Autodesk Fusion 360 part; units mm, degrees
(part 3 of 7)
sketch "Sketch73" plane through (0, 0, 10) normal (0, 0, -1) x (1, 0, 0)
  line L0 (-2, 4.1) -> (0, 4.1)
  line L1 (0, 4.1) -> (0, 5.7)
  arc A0 (8.6603, 8.7) -> (0, 5.7) centre (0, 19.7) ccw
  line L2 (8.6603, 8.7) -> (27.2, 8.7)
  line L3 (27.2, 8.7) -> (27.2, 33.9)
  line L4 (27.2, 33.9) -> (66.7, 33.9)
  line L5 (66.7, 33.9) -> (66.7, 8.7)
  line L6 (66.7, 8.7) -> (85.2397, 8.7)
  arc A1 (93.9, 5.7) -> (85.2397, 8.7) centre (93.9, 19.7) ccw
  line L7 (93.9, 5.7) -> (93.9, 4.1)
  line L8 (93.9, 4.1) -> (95.9, 4.1)
  line L9 (95.9, 4.1) -> (98.4, 4.1)
  line L10 (98.4, 4.1) -> (100.9, 4.1)
  line L11 (100.9, 4.1) -> (126.4, 4.1)
  line L12 (126.4, 4.1) -> (126.4, 25.3)
  arc A2 (126.4, 25.3) -> (116.4, 35.3) centre (116.4, 25.3) ccw
  line L13 (116.4, 35.3) -> (-22.5, 35.3)
  arc A3 (-22.5, 35.3) -> (-32.5, 25.3) centre (-22.5, 25.3) ccw
  line L14 (-32.5, 25.3) -> (-32.5, 4.1)
  line L15 (-32.5, 4.1) -> (-7, 4.1)
  line L16 (-7, 4.1) -> (-4.5, 4.1)
  line L17 (-4.5, 4.1) -> (-2, 4.1)
  line L18 (126.4, 25.3) -> (116.4, 25.3)
  line L19 (116.4, 35.3) -> (116.4, 25.3)
  line L20 (116.4, 25.3) -> (116.4, 4.1)
  line L21 (95.9, -0.9) -> (98.4, -0.9)
  line L22 (95.9, -0.9) -> (113.9, -0.9)
  line L23 (116.4, 2) -> (116.4, 1.2)
  line L24 (118.9, 1.6) -> (118.9, 4.1)
  line L25 (113.9, 1.6) -> (113.9, 4.1)
  line L26 (116.4, 2) -> (116.4, 1.6)
  circle A4 centre (116.4, 1.6) radius 0.4
  circle A5 centre (116.4, 25.3) radius 0.4
  arc A6 (113.9, 1.6) -> (118.9, 1.6) centre (116.4, 1.6) ccw
  circle A7 centre (116.4, 25.3) radius 2.5
  circle A8 centre (116.4, 1.6) radius 2.5
  line L27 (27.2, 4.1) -> (66.7, 4.1)
  line L28 (46.95, 4.1) -> (46.95, -10) construction
  line L29 (46.95, 4.1) -> (46.95, -10) construction
  circle A9 centre (-22.5, 1.6) radius 2.5
  line L30 (-25, 1.6) -> (-25, 4.1)
  line L31 (-7, 4.1) -> (-32.5, 4.1)
  circle A10 centre (-22.5, 25.3) radius 2.5
  line L32 (-20, 1.6) -> (-20, 4.1)
  circle A11 centre (-22.5, 25.3) radius 0.4
  circle A12 centre (-22.5, 1.6) radius 0.4
  point P0 (95.9, -0.9)
  dimension "d491" = 0.8
  dimension "d492" = 0.8
  dimension "d493" = 5
  dimension "d496" = 0.8
  dimension "d497" = 0.8
  constraint coincident L12.end A2.start
  constraint coincident A2.centre L18.end
  constraint coincident A2.end L13.start
  constraint coincident L11 L20.end
  constraint perpendicular L11 L20
  constraint coincident P0 L21.start
  constraint parallel L21 L22
  constraint perpendicular L22 L23
  constraint coincident L11 L24.end
  constraint perpendicular L11 L24
  constraint coincident L11 L25.end
  constraint perpendicular L11 L25
  constraint coincident L26.end A4.centre
  constraint concentric A4 A6
  constraint coincident A4 L23.start
  constraint coincident L23 L26.end
  constraint coincident A4 L23.end
  constraint concentric A6 A8
  constraint coincident L20.end A8
  constraint midpoint L27 L28.start
  constraint perpendicular L2 L28
  constraint symmetric L10.end L28 L15.end
  constraint symmetric L11.end L28 L14.end
  constraint symmetric L24.end L28 L30.end
  constraint symmetric L25.end L28 L32.end
  constraint symmetric L24.start L28 L30.start
  constraint symmetric L25.start L28 L32.start
  constraint symmetric A7 L28 A10
  constraint symmetric A8 L28 A9
  constraint symmetric L29.start L28 L28.start
  constraint symmetric L29.end L28 L28.end
  constraint concentric A10 A11
  constraint concentric A9 A12
  measures "d491" diameter of A4
  measures "d492" diameter of A5
  measures "d493" diameter of A7
  measures "d496" diameter of A11
  measures "d497" diameter of A12
extrude "Extrude58" add sketch "Sketch73" against normal blind 4.6 contours L15 A9 L31 L32 | L15 A9 L30 L31 | A9 | L11 L24 A8 | L11 L25 A8 | A6 A8 | A12 bodies 3
extrude "Extrude59" add sketch "Sketch73" along normal blind 18.4 contours A9 | L18 L19 A5 A7 | L19 L20 A5 A7 | L18 L20 A5 A7 | A6 A8 | A10 bodies 3
sketch "Sketch74" plane through (0, 0, 10) normal (0, 0, -1) x (1, 0, 0)
  circle A0 centre (-22.5, 25.3) radius 2.5
  arc A1 (-20, 1.6) -> (-25, 1.6) centre (-22.5, 1.6) ccw
  line L0 (-20, 1.6) -> (-20, 4.1)
  line L1 (-20, 4.1) -> (-7, 4.1)
  line L2 (-7, 4.1) -> (-4.5, 4.1)
  line L3 (-4.5, 4.1) -> (-2, 4.1)
  line L4 (-2, 4.1) -> (0, 4.1)
  line L5 (0, 4.1) -> (0, 5.7)
  arc A2 (8.6603, 8.7) -> (0, 5.7) centre (0, 19.7) ccw
  line L6 (8.6603, 8.7) -> (27.2, 8.7)
  line L7 (27.2, 8.7) -> (27.2, 33.9)
  line L8 (27.2, 33.9) -> (66.7, 33.9)
  line L9 (66.7, 33.9) -> (66.7, 8.7)
  line L10 (66.7, 8.7) -> (85.2397, 8.7)
  arc A3 (93.9, 5.7) -> (85.2397, 8.7) centre (93.9, 19.7) ccw
  line L11 (93.9, 5.7) -> (93.9, 4.1)
  line L12 (93.9, 4.1) -> (95.9, 4.1)
  line L13 (95.9, 4.1) -> (98.4, 4.1)
  line L14 (98.4, 4.1) -> (100.9, 4.1)
  line L15 (100.9, 4.1) -> (113.9, 4.1)
  line L16 (113.9, 4.1) -> (113.9, 1.6)
  arc A4 (118.9, 1.6) -> (113.9, 1.6) centre (116.4, 1.6) ccw
  line L17 (118.9, 1.6) -> (118.9, 4.1)
  line L18 (118.9, 4.1) -> (126.4, 4.1)
  line L19 (126.4, 4.1) -> (126.4, 25.3)
  arc A5 (126.4, 25.3) -> (116.4, 35.3) centre (116.4, 25.3) ccw
  line L20 (116.4, 35.3) -> (-22.5, 35.3)
  arc A6 (-22.5, 35.3) -> (-32.5, 25.3) centre (-22.5, 25.3) ccw
  line L21 (-32.5, 25.3) -> (-32.5, 4.1)
  line L22 (-32.5, 4.1) -> (-25, 4.1)
  line L23 (-25, 4.1) -> (-25, 1.6)
  circle A7 centre (116.4, 25.3) radius 2.5
  line L24 (79.9, 19.7) -> (79.9, 15.7)
  line L25 (79.9, 19.7) -> (79.9, 23.7)
  line L26 (79.9, 19.7) -> (66.7, 19.7)
  line L27 (66.7, 19.7) -> (66.7, 15.7)
  line L28 (66.7, 19.7) -> (66.7, 23.7)
  line L29 (66.7, 15.7) -> (81.7498, 15.7)
  line L30 (66.7, 23.7) -> (82, 23.7)
  line L31 (82, 23.7) -> (79.9, 23.7)
  line L32 (79.9, 23.7) -> (12.6632, 23.7)
  line L33 (12.6632, 15.7) -> (79.9, 15.7)
  line L34 (12.6632, 15.7) -> (9.5, 15.7)
  line L35 (9.5, 15.7) -> (9.5, 23.7)
  line L36 (9.5, 23.7) -> (12.6632, 23.7)
  line L37 (81.7498, 15.7) -> (83.7784, 15.7)
  line L38 (83.7784, 15.7) -> (83.7784, 23.7)
  line L39 (83.7784, 23.7) -> (82, 23.7)
  point P0 (79.9, 19.7)
  dimension "d500" = 4
  dimension "d501" = 4
  dimension "d502" = 4
  dimension "d503" = 4
  dimension "d504" = 180
  dimension "d505" = 8
  constraint coincident P0 L24.start
  constraint vertical L24
  constraint parallel L24 L25
  constraint horizontal L26
  constraint coincident L9 L26.end
  constraint perpendicular L26 L27
  constraint perpendicular L26 L28
  constraint perpendicular L24 L29
  constraint perpendicular L9 L30
  constraint perpendicular L32 L35
  constraint parallel L29 L37
  constraint perpendicular L30 L38
  constraint perpendicular L38 L39
  measures "d500" distance of P0 L24.end
  measures "d501" distance of P0 L25.end
  measures "d502" distance of L26.end L27.end
  measures "d503" distance of L26.end L28.end
  measures "d504" angle of L31 L32
  measures "d505" distance of L32.end L33.start
extrude "Extrude60" cut sketch "Sketch74" against normal blind 4.6 contours A2 L7 L32 L33 | A2 L32 L33 L34 L35 L36 | L9 L25 L26 L28 L30 L32 | L9 L24 L26 L27 L29 L33 | A3 L25 L30 L31 | A3 L24 L29 | A3 L29 L30 L31 L37 L38 L39 bodies 3
sketch "Sketch76" plane through (0, 0, 14.6) normal (0, 0, -1) x (1, 0, 0)
  line L0 (113.9, 1.6) -> (113.9, 4.1)
  line L1 (113.9, 4.1) -> (100.9, 4.1)
  line L2 (100.9, 4.1) -> (100.9, 1.6)
  arc A0 (98.4, -0.9) -> (100.9, 1.6) centre (98.4, 1.6) ccw
  line L3 (98.4, -0.9) -> (95.9, -0.9)
  line L4 (95.9, -0.9) -> (95.9, -77.2)
  line L5 (95.9, -77.2) -> (75.9, -77.2)
  line L6 (75.9, -77.2) -> (75.9, -85.1)
  line L7 (75.9, -85.1) -> (106.4, -85.1)
  arc A1 (106.4, -85.1) -> (126.4, -65.1) centre (106.4, -65.1) ccw
  line L8 (126.4, -65.1) -> (126.4, 4.1)
  line L9 (126.4, 4.1) -> (118.9, 4.1)
  line L10 (118.9, 4.1) -> (118.9, 1.6)
  arc A2 (113.9, 1.6) -> (118.9, 1.6) centre (116.4, 1.6) ccw
  line L11 (107.65, -43.95) -> (107.65, -38.95)
  line L12 (107.65, -38.95) -> (112.65, -38.95)
  line L13 (112.65, -38.95) -> (112.65, -43.95)
  line L14 (112.65, -43.95) -> (107.65, -43.95)
  circle A3 centre (117.6453, -56.4453) radius 2.85
  circle A4 centre (102.6547, -56.4453) radius 2.85
  line L15 (113.3329, -38.8299) -> (112.9477, -38.4448)
  line L16 (112.9477, -38.4448) -> (114.6448, -36.7477)
  line L17 (114.6448, -36.7477) -> (115.0299, -37.1329)
  arc A5 (122.2, -39.2591) -> (115.0299, -37.1329) centre (117.65, -41.45) ccw
  line L18 (122.2, -39.2591) -> (122.2, -43.6409)
  arc A6 (113.1, -43.6409) -> (122.2, -43.6409) centre (117.65, -41.45) ccw
  line L19 (113.1, -43.6409) -> (113.1, -39.2591)
  arc A7 (113.3329, -38.8299) -> (113.1, -39.2591) centre (117.65, -41.45) ccw
  line L20 (106.9671, -44.0701) -> (107.3523, -44.4552)
  line L21 (107.3523, -44.4552) -> (105.6552, -46.1523)
  line L22 (105.6552, -46.1523) -> (105.2701, -45.7671)
  arc A8 (98.115, -43.6717) -> (105.2701, -45.7671) centre (102.65, -41.45) ccw
  line L23 (98.115, -43.6717) -> (98.0852, -39.29)
  arc A9 (107.185, -39.2283) -> (98.0852, -39.29) centre (102.65, -41.45) ccw
  line L24 (107.185, -39.2283) -> (107.2148, -43.61)
  arc A10 (106.9671, -44.0701) -> (107.2148, -43.61) centre (102.65, -41.45) ccw
  line L25 (112.7701, -44.6329) -> (113.1552, -44.2477)
  line L26 (113.1552, -44.2477) -> (114.8523, -45.9448)
  line L27 (114.8523, -45.9448) -> (114.4671, -46.3299)
  arc A11 (112.3364, -53.5022) -> (114.4671, -46.3299) centre (110.15, -48.95) ccw
  line L28 (112.3364, -53.5022) -> (112.3364, -53.5)
  line L29 (112.3364, -53.5) -> (107.9591, -53.5)
  arc A12 (107.9591, -44.4) -> (107.9591, -53.5) centre (110.15, -48.95) ccw
  line L30 (107.9591, -44.4) -> (112.3409, -44.4)
  arc A13 (112.7701, -44.6329) -> (112.3409, -44.4) centre (110.15, -48.95) ccw
  line L31 (107.5299, -38.2671) -> (107.1448, -38.6523)
  line L32 (107.1448, -38.6523) -> (105.4477, -36.9552)
  line L33 (105.4477, -36.9552) -> (105.8329, -36.5701)
  arc A14 (107.9591, -29.4) -> (105.8329, -36.5701) centre (110.15, -33.95) ccw
  line L34 (107.9591, -29.4) -> (112.3409, -29.4)
  arc A15 (112.3409, -38.5) -> (112.3409, -29.4) centre (110.15, -33.95) ccw
  line L35 (112.3409, -38.5) -> (107.9591, -38.5)
  arc A16 (107.5299, -38.2671) -> (107.9591, -38.5) centre (110.15, -33.95) ccw
  circle A17 centre (110.15, -62.1) radius 2.5
  circle A18 centre (110.2363, -20.8316) radius 2.5
  circle A19 centre (117.6453, -56.4453) radius 5
  circle A20 centre (102.6547, -56.4453) radius 5
  dimension "d509" = 10
  dimension "d510" = 10
  constraint concentric A3 A19
  constraint concentric A4 A20
  measures "d509" diameter of A19
  measures "d510" diameter of A20
extrude "Extrude61" cut sketch "Sketch76" against normal blind 0.5 contours A19 | A20 bodies 3
sketch "Sketch77" plane through (0, 0, 10) normal (0, 0, -1) x (1, 0, 0)
  line L0 (66.7, 23.7) -> (80.4836, 23.7)
  arc A0 (93.9, 5.7) -> (80.4836, 23.7) centre (93.9, 19.7) ccw
  line L1 (93.9, 5.7) -> (93.9, 4.1)
  line L2 (93.9, 4.1) -> (95.9, 4.1)
  line L3 (95.9, 4.1) -> (98.4, 4.1)
  line L4 (98.4, 4.1) -> (100.9, 4.1)
  line L5 (100.9, 4.1) -> (113.9, 4.1)
  line L6 (113.9, 4.1) -> (113.9, 1.6)
  arc A1 (118.9, 1.6) -> (113.9, 1.6) centre (116.4, 1.6) ccw
  line L7 (118.9, 1.6) -> (118.9, 4.1)
  line L8 (118.9, 4.1) -> (126.4, 4.1)
  line L9 (126.4, 4.1) -> (126.4, 25.3)
  arc A2 (126.4, 25.3) -> (116.4, 35.3) centre (116.4, 25.3) ccw
  line L10 (116.4, 35.3) -> (-22.5, 35.3)
  arc A3 (-22.5, 35.3) -> (-32.5, 25.3) centre (-22.5, 25.3) ccw
  line L11 (-32.5, 25.3) -> (-32.5, 4.1)
  line L12 (-32.5, 4.1) -> (-25, 4.1)
  line L13 (-25, 4.1) -> (-25, 1.6)
  arc A4 (-20, 1.6) -> (-25, 1.6) centre (-22.5, 1.6) ccw
  line L14 (-20, 1.6) -> (-20, 4.1)
  line L15 (-20, 4.1) -> (-7, 4.1)
  line L16 (-7, 4.1) -> (-4.5, 4.1)
  line L17 (-4.5, 4.1) -> (-2, 4.1)
  line L18 (-2, 4.1) -> (0, 4.1)
  line L19 (0, 4.1) -> (0, 5.7)
  arc A5 (13.4164, 23.7) -> (0, 5.7) centre (0, 19.7) ccw
  line L20 (13.4164, 23.7) -> (27.2, 23.7)
  line L21 (27.2, 23.7) -> (27.2, 33.9)
  line L22 (27.2, 33.9) -> (66.7, 33.9)
  line L23 (66.7, 33.9) -> (66.7, 23.7)
  circle A6 centre (-22.5, 25.3) radius 2.5
  circle A7 centre (116.4, 25.3) radius 2.5
  line L24 (-22.5, 1.6) -> (-22.5, 25.3)
  line L25 (-22.5, 24.9) -> (-23, 24.9)
  line L26 (-23, 24.9) -> (-22, 24.9)
  line L27 (-22.5, 2) -> (-23, 2)
  line L28 (-22.5, 2) -> (-22, 2)
  line L29 (-22, 2) -> (-23, 2)
  line L30 (-23, 2) -> (-23, 24.9)
  line L31 (-23, 24.9) -> (-22, 24.9)
  line L32 (-22, 24.9) -> (-22, 2)
  line L33 (27.2, 4.5) -> (66.7, 4.5)
  line L34 (27.2, 4.1) -> (66.7, 4.1)
  line L35 (46.95, 4.5) -> (46.95, -16.4696) construction
  line L36 (116.4, 2) -> (116.9, 2)
  line L37 (116.9, 2) -> (116.9, 24.9)
  line L38 (116.4, 2) -> (115.9, 2)
  line L39 (116.9, 24.9) -> (115.9, 24.9)
  line L40 (115.9, 24.9) -> (115.9, 2)
  dimension "d513" = 1
  dimension "d514" = 0.5
  constraint coincident A4.centre L24.start
  constraint coincident A3.centre A6.centre
  constraint coincident L24 L25.start
  constraint perpendicular L24 L25
  constraint horizontal L26
  constraint coincident L24 L27.start
  constraint perpendicular L24 L27
  constraint perpendicular L24 L28
  constraint horizontal L29
  constraint vertical L30
  constraint horizontal L31
  constraint vertical L32
  constraint midpoint L33 L35.start
  constraint perpendicular L34 L35
  constraint symmetric L25.end L35 L37.end
  constraint symmetric L27.start L35 L36.start
  constraint symmetric L27.end L35 L36.end
  constraint symmetric L28.end L35 L38.end
  constraint symmetric L26.end L35 L39.end
  measures "d513" distance of L25.end L26.end
  measures "d514" distance of L27.start L27.end
extrude "Extrude63" add sketch "Sketch77" along normal blind 4 contours A1 A7 L37 L40 | A4 A6 L24 L32 | A4 A6 L24 L30 bodies 3
sketch "Sketch78" plane through (0, 0, 14.6) normal (0, 0, -1) x (1, 0, 0)
  line L0 (-25, 1.6) -> (-25, 4.1)
  line L1 (-25, 4.1) -> (-32.5, 4.1)
  line L2 (-32.5, 4.1) -> (-32.5, -25.2)
  line L3 (-32.5, -25.2) -> (-32.5, -65.1)
  arc A0 (-32.5, -65.1) -> (-12.5, -85.1) centre (-12.5, -65.1) ccw
  line L4 (-12.5, -85.1) -> (-2, -85.1)
  line L5 (-2, -85.1) -> (-2, -0.9)
  line L6 (-2, -0.9) -> (-4.5, -0.9)
  arc A1 (-7, 1.6) -> (-4.5, -0.9) centre (-4.5, 1.6) ccw
  line L7 (-7, 1.6) -> (-7, 4.1)
  line L8 (-7, 4.1) -> (-20, 4.1)
  line L9 (-20, 4.1) -> (-20, 1.6)
  arc A2 (-25, 1.6) -> (-20, 1.6) centre (-22.5, 1.6) ccw
  arc A3 (-9.5307, -48.3426) -> (-9.5307, -34.5574) centre (-10.1676, -41.45) ccw
  arc A4 (-22.9827, -48.1827) -> (-9.5307, -48.3426) centre (-16.25, -47.7) ccw
  arc A5 (-22.9827, -34.7173) -> (-22.9827, -48.1827) centre (-22.5, -41.45) ccw
  arc A6 (-9.5307, -34.5574) -> (-22.9827, -34.7173) centre (-16.25, -35.2) ccw
  circle A7 centre (-16.25, -62.1) radius 2.5
  circle A8 centre (-16.1626, -20.3028) radius 2.5
  circle A9 centre (-22.5, 1.6) radius 0.4
  circle A10 centre (-22.5, 1.6) radius 0.4
  circle A11 centre (-4.5, 1.6) radius 0.4
  line L10 (-22.5, 1.2) -> (-4.5, 1.2)
  line L11 (-4.5, 2) -> (-22.5, 2)
  line L12 (-4.5, 1.2) -> (-4.5, 2)
  line L13 (-22.5, 1.2) -> (-22.5, 2)
  line L14 (46.95, 4.5) -> (46.95, -16.4696)
  line L15 (98.4, 2) -> (116.4, 2)
  line L16 (98.4, 1.2) -> (98.4, 2)
  line L17 (116.4, 1.2) -> (98.4, 1.2)
  line L18 (116.4, 1.2) -> (116.4, 2)
  circle A12 centre (-22.5, 1.6) radius 0.4
  circle A13 centre (-4.5, 1.6) radius 0.4
  circle A14 centre (98.4, 1.6) radius 0.4
  circle A15 centre (98.4, 1.6) radius 0.4
  circle A16 centre (116.4, 1.6) radius 0.4
  point P0 (-4.9, 1.6)
  point P1 (116.4, 1.6)
  constraint coincident A9 L10.start
  constraint coincident A10 L10.start
  constraint coincident A11 L10.end
  constraint coincident A11 L11.start
  constraint coincident A9 L11.end
  constraint perpendicular L10 L12
  constraint perpendicular L11 L13
  constraint symmetric L10.start L14 L17.start
  constraint symmetric L10.end L14 L16.start
  constraint symmetric L11.start L14 L15.start
  constraint symmetric L11.end L14 L15.end
  constraint concentric A10 A12
  constraint concentric A11 A13
  constraint coincident A13 P0
  constraint concentric A14 A15
  constraint coincident P1 A16.centre
extrude "Extrude64" add sketch "Sketch78" along normal blind 8.6 contours A1 L7 L9 A2 L10 L11 | L15 L17 A14 A15 A16 bodies 3
extrude "Extrude65" add 2 faces at (-15.6667, -2.7, 14.6) (109.5667, -2.7, 14.6) along direction (0, 0, -1) blind 4.6 on bodies 3 bodies 3
sketch "Sketch79" plane through (0, 0, 10) normal (0, 0, -1) x (1, 0, 0)
  arc A0 (70.9, -81.15) -> (75.9, -81.15) centre (73.4, -81.15) ccw
  line L0 (70.9, -81.15) -> (70.9, -77.2)
  line L1 (70.9, -77.2) -> (47.4908, -77.2)
  arc A1 (46.4092, -77.2) -> (47.4908, -77.2) centre (46.95, -80.1) ccw
  line L2 (46.4092, -77.2) -> (10.5, -77.2)
  line L3 (10.5, -77.2) -> (10.5, -81.15)
  arc A2 (5.5, -81.15) -> (10.5, -81.15) centre (8, -81.15) ccw
  line L4 (5.5, -81.15) -> (5.5, -77.2)
  line L5 (5.5, -77.2) -> (-2, -77.2)
  line L6 (-2, -77.2) -> (-2, -85.1)
  line L7 (-2, -85.1) -> (75.9, -85.1)
  line L8 (75.9, -85.1) -> (75.9, -81.15)
  line L9 (46.95, -80.1) -> (73.4, -80.1)
  line L10 (46.95, -80.1) -> (23, -80.1)
  line L11 (73.4, -80.1) -> (73.4, -81.15)
  line L12 (20.5, -80.75) -> (20.5, -81.15)
  line L13 (20.5, -81.15) -> (20.1, -81.15)
  line L14 (20.5, -81.15) -> (20.9, -81.15)
  line L15 (20.5, -81.15) -> (20.1, -81.15)
  line L16 (23, -81.15) -> (23, -77.2)
  line L17 (18, -81.15) -> (18, -77.2)
  line L18 (18, -77.2) -> (23, -77.2)
  circle A3 centre (20.5, -81.15) radius 0.4
  line L19 (8, -81.15) -> (18, -81.15)
  line L20 (20.1, -81.15) -> (20.5, -81.15)
  arc A4 (18, -81.15) -> (23, -81.15) centre (20.5, -81.15) ccw
  dimension "d527" = 2.5
  dimension "d528" = 2.5
  dimension "d529" = 0.8
  constraint coincident A1.centre L9.start
  constraint horizontal L9
  constraint parallel L9 L10
  constraint coincident A0.centre L11.end
  constraint perpendicular L9 L11
  constraint perpendicular L10 L12
  constraint coincident A2.centre L19.start
  constraint perpendicular L12 L13
  constraint perpendicular L12 L14
  constraint coincident L12.end L13.start
  constraint coincident L2 L16.end
  constraint tangent L16 A4
  constraint perpendicular L2 L16
  constraint coincident L2 L17.end
  constraint tangent L17 A4
  constraint concentric A3 A4
  constraint coincident A3 L14.end
  constraint coincident A3 L13.end
  constraint collinear L19 L20
  constraint coincident L16 L10.end
  constraint coincident A3 L12.start
  measures "d527" distance of L12.end L17.start
  measures "d528" distance of L12.end L16.start
  measures "d529" diameter of A3
extrude "Extrude66" add sketch "Sketch79" along normal blind 6 contours L2 L16 L17 L18 A4 bodies 3
sketch "Sketch80" plane through (0, 0, 4) normal (0, 0, -1) x (1, 0, 0)
  circle A0 centre (20.5, -81.15) radius 0.4
  circle A1 centre (73.4, -81.15) radius 0.4
  circle A2 centre (8, -81.15) radius 0.4
  circle A3 centre (-4.5, 1.6) radius 0.4
  circle A4 centre (98.4, 1.6) radius 0.4
  line L0 (95.9, 4.1) -> (93.9, 4.1)
  line L1 (93.9, 4.1) -> (93.9, -75.1)
  line L2 (93.9, -75.1) -> (0, -75.1)
  line L3 (0, -75.1) -> (0, 4.1)
  line L4 (0, 4.1) -> (-4.5, 4.1)
  line L5 (-4.5, 4.1) -> (-7, 4.1)
  line L6 (-7, 4.1) -> (-7, 1.6)
  arc A5 (-7, 1.6) -> (-4.5, -0.9) centre (-4.5, 1.6) ccw
  line L7 (-4.5, -0.9) -> (-2, -0.9)
  line L8 (-2, -0.9) -> (-2, -77.2)
  line L9 (-2, -77.2) -> (5.5, -77.2)
  line L10 (5.5, -77.2) -> (5.5, -81.15)
  arc A6 (5.5, -81.15) -> (10.5, -81.15) centre (8, -81.15) ccw
  line L11 (10.5, -81.15) -> (10.5, -77.2)
  line L12 (10.5, -77.2) -> (18, -77.2)
  line L13 (18, -77.2) -> (18, -81.15)
  arc A7 (18, -81.15) -> (23, -81.15) centre (20.5, -81.15) ccw
  line L14 (23, -81.15) -> (23, -77.2)
  line L15 (23, -77.2) -> (46.4092, -77.2)
  arc A8 (47.4908, -77.2) -> (46.4092, -77.2) centre (46.95, -80.1) ccw
  line L16 (47.4908, -77.2) -> (70.9, -77.2)
  line L17 (70.9, -77.2) -> (70.9, -81.15)
  arc A9 (70.9, -81.15) -> (75.9, -81.15) centre (73.4, -81.15) ccw
  line L18 (75.9, -81.15) -> (75.9, -77.2)
  line L19 (75.9, -77.2) -> (95.9, -77.2)
  line L20 (95.9, -77.2) -> (95.9, -0.9)
  line L21 (95.9, -0.9) -> (98.4, -0.9)
  arc A10 (98.4, -0.9) -> (100.9, 1.6) centre (98.4, 1.6) ccw
  line L22 (100.9, 1.6) -> (100.9, 4.1)
  line L23 (100.9, 4.1) -> (98.4, 4.1)
  line L24 (98.4, 4.1) -> (95.9, 4.1)
  circle A11 centre (20.5, -81.15) radius 2.5
  constraint concentric A0 A11
  constraint coincident L13.end A11
extrude "Extrude67" add sketch "Sketch80" along normal blind 12.4 contours A7 A11 bodies 3
sketch "Sketch81" plane through (0, 0, 2.4) normal (0, 0, -1) x (1, 0, 0)
  circle A0 centre (84.4, -5) radius 2.5
  circle A1 centre (98.4, 1.6) radius 1
  circle A2 centre (73.4, -81.15) radius 1
  circle A3 centre (-4.5, 1.6) radius 1
  circle A4 centre (80.15, -44.4) radius 2.5
  circle A5 centre (8, -81.15) radius 1
  circle A6 centre (10.06, -44.3) radius 2.5
  line L0 (-2, -83.65) -> (95.9, -83.65)
  line L1 (95.9, -83.65) -> (95.9, -3.65)
  line L2 (95.9, -3.65) -> (100.9, -3.65)
  line L3 (100.9, -3.65) -> (100.9, 4.1)
  line L4 (100.9, 4.1) -> (-7, 4.1)
  line L5 (-7, 4.1) -> (-7, -3.65)
  line L6 (-7, -3.65) -> (-2, -3.65)
  line L7 (-2, -3.65) -> (-2, -83.65)
  circle A7 centre (20.5, -81.15) radius 0.4
  line L8 (18, -77.2) -> (18, -81.15)
  line L9 (20.5, -81.15) -> (16.5, -81.15)
  line L10 (20.5, -81.15) -> (24.5, -81.15)
  line L11 (46.4092, -77.2) -> (23, -77.2)
  line L12 (24.5, -81.15) -> (24.5, -77.2)
  line L13 (10.5, -77.2) -> (18, -77.2)
  line L14 (24.5, -77.2) -> (16.5, -77.2)
  line L15 (16.5, -77.2) -> (16.5, -83.65)
  line L16 (16.5, -83.65) -> (24.5, -83.65)
  line L17 (24.5, -83.65) -> (24.5, -81.15)
  dimension "d534" = 4
  dimension "d535" = 4
  constraint coincident A7.centre L9.start
  constraint perpendicular L8 L9
  constraint parallel L9 L10
  constraint coincident L11 L12.end
  constraint perpendicular L10 L12
  constraint coincident L13 L14.end
  constraint coincident L0 L15.end
  constraint perpendicular L0 L15
  constraint coincident L0 L16.end
  constraint perpendicular L12 L16
  measures "d534" distance of A7.centre L9.end
  measures "d535" distance of A7.centre L10.end
extrude "Extrude68" cut sketch "Sketch81" against normal blind 1.6 contours L0 A7 L9 L10 L15 L16 L17 | L8 L9 L13 L14 L15 | A7 L8 L9 L10 L11 L12 L14 | A7 L9 L10 | A7 L9 L10 bodies 8
sketch "Sketch82" plane through (0, 0, 14.6) normal (0, 0, -1) x (1, 0, 0)
  circle A0 centre (117.6453, -56.4453) radius 5
  circle A1 centre (102.6547, -56.4453) radius 5
  line L0 (113.9322, 1.2) -> (100.8678, 1.2)
  arc A2 (98.4, -0.9) -> (100.8678, 1.2) centre (98.4, 1.6) ccw
  line L1 (98.4, -0.9) -> (95.9, -0.9)
  line L2 (95.9, -0.9) -> (95.9, -77.2)
  line L3 (95.9, -77.2) -> (75.9, -77.2)
  line L4 (75.9, -77.2) -> (75.9, -85.1)
  line L5 (75.9, -85.1) -> (106.4, -85.1)
  arc A3 (106.4, -85.1) -> (126.4, -65.1) centre (106.4, -65.1) ccw
  line L6 (126.4, -65.1) -> (126.4, 4.1)
  line L7 (126.4, 4.1) -> (118.9, 4.1)
  line L8 (118.9, 4.1) -> (118.9, 1.6)
  arc A4 (113.9322, 1.2) -> (118.9, 1.6) centre (116.4, 1.6) ccw
  line L9 (107.65, -43.95) -> (107.65, -38.95)
  line L10 (107.65, -38.95) -> (112.65, -38.95)
  line L11 (112.65, -38.95) -> (112.65, -43.95)
  line L12 (112.65, -43.95) -> (107.65, -43.95)
  line L13 (113.3329, -38.8299) -> (112.9477, -38.4448)
  line L14 (112.9477, -38.4448) -> (114.6448, -36.7477)
  line L15 (114.6448, -36.7477) -> (115.0299, -37.1329)
  arc A5 (122.2, -39.2591) -> (115.0299, -37.1329) centre (117.65, -41.45) ccw
  line L16 (122.2, -39.2591) -> (122.2, -43.6409)
  arc A6 (113.1, -43.6409) -> (122.2, -43.6409) centre (117.65, -41.45) ccw
  line L17 (113.1, -43.6409) -> (113.1, -39.2591)
  arc A7 (113.3329, -38.8299) -> (113.1, -39.2591) centre (117.65, -41.45) ccw
  line L18 (106.9671, -44.0701) -> (107.3523, -44.4552)
  line L19 (107.3523, -44.4552) -> (105.6552, -46.1523)
  line L20 (105.6552, -46.1523) -> (105.2701, -45.7671)
  arc A8 (98.115, -43.6717) -> (105.2701, -45.7671) centre (102.65, -41.45) ccw
  line L21 (98.115, -43.6717) -> (98.0852, -39.29)
  arc A9 (107.185, -39.2283) -> (98.0852, -39.29) centre (102.65, -41.45) ccw
  line L22 (107.185, -39.2283) -> (107.2148, -43.61)
  arc A10 (106.9671, -44.0701) -> (107.2148, -43.61) centre (102.65, -41.45) ccw
  line L23 (112.7701, -44.6329) -> (113.1552, -44.2477)
  line L24 (113.1552, -44.2477) -> (114.8523, -45.9448)
  line L25 (114.8523, -45.9448) -> (114.4671, -46.3299)
  arc A11 (112.3364, -53.5022) -> (114.4671, -46.3299) centre (110.15, -48.95) ccw
  line L26 (112.3364, -53.5022) -> (112.3364, -53.5)
  line L27 (112.3364, -53.5) -> (107.9591, -53.5)
  arc A12 (107.9591, -44.4) -> (107.9591, -53.5) centre (110.15, -48.95) ccw
  line L28 (107.9591, -44.4) -> (112.3409, -44.4)
  arc A13 (112.7701, -44.6329) -> (112.3409, -44.4) centre (110.15, -48.95) ccw
  line L29 (107.5299, -38.2671) -> (107.1448, -38.6523)
  line L30 (107.1448, -38.6523) -> (105.4477, -36.9552)
  line L31 (105.4477, -36.9552) -> (105.8329, -36.5701)
  arc A14 (107.9591, -29.4) -> (105.8329, -36.5701) centre (110.15, -33.95) ccw
  line L32 (107.9591, -29.4) -> (112.3409, -29.4)
  arc A15 (112.3409, -38.5) -> (112.3409, -29.4) centre (110.15, -33.95) ccw
  line L33 (112.3409, -38.5) -> (107.9591, -38.5)
  arc A16 (107.5299, -38.2671) -> (107.9591, -38.5) centre (110.15, -33.95) ccw
  circle A17 centre (110.15, -62.1) radius 2.5
  circle A18 centre (110.2363, -20.8316) radius 2.5
  line L34 (126.4, 4.1) -> (125.4, 4.1)
  line L35 (125.4, 4.1) -> (125.4, -25.9)
  line L36 (125.4, -25.9) -> (124.4, -25.9)
  line L37 (124.4, -25.9) -> (124.4, 4.1)
  line L38 (124.4, -25.9) -> (124.4, -24.9)
  line L39 (95.9, -24.9) -> (95.9, -25.9)
  line L40 (124.4, 4.1) -> (125.4, 4.1)
  line L41 (95.9, -24.9) -> (100.9, -24.9)
  line L42 (100.9, -24.9) -> (101.9, -24.9)
  line L43 (118.9, -24.9) -> (119.9, -24.9)
  line L44 (119.9, -24.9) -> (119.9, 4.1)
  line L45 (118.9, -24.9) -> (118.9, 4.1)
  line L46 (101.9, -24.9) -> (101.9, 1.2)
  line L47 (100.9, -24.9) -> (100.8678, 1.2)
  line L48 (95.9, -24.9) -> (95.9, -19.9)
  line L49 (95.9, -19.9) -> (95.9, -18.9)
  line L50 (95.9, -18.9) -> (95.9, -13.9)
  line L51 (95.9, -13.9) -> (95.9, -12.9)
  line L52 (95.9, -12.9) -> (95.9, -7.9)
  line L53 (95.9, -7.9) -> (95.9, -6.9)
  line L54 (95.9, -6.9) -> (95.9, -1.9)
  line L55 (95.9, -1.9) -> (95.9, -0.9)
  line L56 (95.9, -1.9) -> (124.4, -1.9)
  line L57 (95.9, -0.9) -> (124.4, -0.9)
  line L58 (27.2, 4.5) -> (66.7, 4.5)
  line L59 (46.95, 4.5) -> (46.95, -22.9595) construction
  line L60 (-2, -6.9) -> (-2, -1.9)
  line L61 (-2, -6.9) -> (-30.5, -6.9)
  line L62 (-2, -0.9) -> (-30.5, -0.9)
  line L63 (-2, -18.9) -> (-2, -13.9)
  arc A19 (-25, 1.6) -> (-20.0322, 1.2) centre (-22.5, 1.6) ccw
  line L64 (-2, -1.9) -> (-30.5, -1.9)
  circle A20 centre (-16.3363, -20.8316) radius 2.5
  arc A21 (-6.9678, 1.2) -> (-4.5, -0.9) centre (-4.5, 1.6) ccw
  line L65 (-2, -19.9) -> (-2, -18.9)
  line L66 (-2, -12.9) -> (-2, -7.9)
  line L67 (-31.5, -25.9) -> (-25, -25.9)
  line L68 (-31.5, -25.9) -> (-30.5, -25.9)
  line L69 (-2, -7.9) -> (-2, -6.9)
  line L70 (-2, -13.9) -> (-2, -12.9)
  line L71 (-2, -24.9) -> (-2, -19.9)
  line L72 (-8, -24.9) -> (-8, 1.2)
  line L73 (-20.0322, 1.2) -> (-6.9678, 1.2)
  line L74 (-4.5, -0.9) -> (-2, -0.9)
  line L75 (-31.5, 4.1) -> (-31.5, -25.9)
  line L76 (-32.5, 4.1) -> (-25, 4.1)
  line L77 (-30.5, 4.1) -> (-31.5, 4.1)
  line L78 (-25, 4.1) -> (-25, 1.6)
  line L79 (-25, -24.9) -> (-25, 4.1)
  line L80 (-7, -24.9) -> (-6.9678, 1.2)
  line L81 (-2, -24.9) -> (-7, -24.9)
  line L82 (-2, -1.9) -> (-2, -0.9)
  line L83 (-2, -7.9) -> (-30.5, -7.9)
  line L84 (-2, -24.9) -> (-2, -25.9)
  line L85 (-26, -24.9) -> (-26, 4.1)
  line L86 (-25, -24.9) -> (-26, -24.9)
  line L87 (-32.5, 4.1) -> (-31.5, 4.1)
  line L88 (-7, -24.9) -> (-8, -24.9)
  line L89 (-30.5, -25.9) -> (-30.5, 4.1)
  line L90 (-30.5, -25.9) -> (-30.5, -24.9)
  line L91 (-25, -19.9) -> (-30.5, -19.9)
  line L92 (-20, -13.9) -> (-20, 1.2)
  line L93 (-25, -18.9) -> (-30.5, -18.9)
  line L94 (-19, -13.9) -> (-19, 1.2)
  line L95 (-25, -24.9) -> (-25, -25.9)
  line L96 (-30.5, -24.9) -> (-25, -24.9)
  line L97 (-2, -12.9) -> (-8, -12.9)
  line L98 (-13, -12.9) -> (-30.5, -12.9)
  line L99 (-2, -13.9) -> (-8, -13.9)
  line L100 (-13, -13.9) -> (-30.5, -13.9)
  line L101 (-2, -18.9) -> (-8, -18.9)
  line L102 (-14.7492, -18.9) -> (-17.9235, -18.9)
  line L103 (-2, -19.9) -> (-8, -19.9)
  line L104 (-14, -19.9) -> (-18.6563, -19.9)
  line L105 (-2, -25.9) -> (-8, -25.9)
  line L106 (-8, -25.9) -> (-8, -24.9)
  line L107 (-8, -24.9) -> (-2, -24.9)
  line L108 (-13, -13.9) -> (-13, 1.2)
  line L109 (-14, -21.7213) -> (-14, -19.9)
  line L110 (-14, -13.9) -> (-14, 1.2)
  line L111 (95.9, -19.9) -> (101.9, -19.9)
  line L112 (95.9, -13.9) -> (101.9, -13.9)
  line L113 (112.9, -13.9) -> (124.4, -13.9)
  line L114 (106.9, -7.9) -> (106.9, 1.2)
  line L115 (107.9, -7.9) -> (107.9, 1.2)
  line L116 (112.9, -12.9) -> (124.4, -12.9)
  line L117 (107.9, -19.9418) -> (107.9, -19.9)
  line L118 (95.9, -12.9) -> (101.9, -12.9)
  line L119 (95.9, -7.9) -> (101.9, -7.9)
  line L120 (106.9, -7.9) -> (124.4, -7.9)
  line L121 (95.9, -6.9) -> (101.9, -6.9)
  line L122 (106.9, -6.9) -> (124.4, -6.9)
  line L123 (112.9, -13.9) -> (112.9, 1.2)
  line L124 (113.9, -13.9) -> (113.9, 1.2)
  line L125 (95.9, -18.9) -> (101.9, -18.9)
  line L126 (108.6492, -18.9) -> (111.8235, -18.9)
  line L127 (118.9, -18.9) -> (124.4, -18.9)
  line L128 (107.9, -19.9) -> (112.5563, -19.9)
  line L129 (118.9, -19.9) -> (124.4, -19.9)
  line L130 (101.9, -24.9) -> (101.9, -25.9)
  line L131 (118.9, -24.9) -> (118.9, -25.9)
  line L132 (125.4, -25.9) -> (118.9, -25.9)
  line L133 (101.9, -25.9) -> (95.9, -25.9)
  line L134 (124.4, -24.9) -> (118.9, -24.9)
  line L135 (101.9, -24.9) -> (95.9, -24.9)
  dimension "d538" = 1
  dimension "d539" = 30
  dimension "d540" = 1
  dimension "d541" = 1
  dimension "d542" = 5
  dimension "d543" = 1
  dimension "d549" = 1
  dimension "d550" = 180
  dimension "d551" = 5
  dimension "d552" = 1
  dimension "d553" = 5
  dimension "d554" = 1
  dimension "d555" = 5
  dimension "d556" = 1
  dimension "d557" = 5
  constraint coincident L6.end L7.start
  constraint perpendicular L6 L34
  constraint perpendicular L34 L35
  constraint coincident L2 L39.end
  constraint perpendicular L2 L132
  constraint perpendicular L35 L36
  constraint coincident L7 L37.end
  constraint perpendicular L7 L37
  constraint perpendicular L36 L38
  constraint coincident L2 L39.start
  constraint perpendicular L2 L134
  constraint perpendicular L39 L41
  constraint perpendicular L6 L42
  constraint parallel L43 L134
  constraint coincident L7 L44.end
  constraint perpendicular L7 L44
  constraint coincident L7 L8.start
  constraint coincident L0 L124.end
  constraint coincident L0 L123.end
  constraint coincident L0 L115.end
  constraint perpendicular L0 L117
  constraint coincident L0 L114.end
  constraint coincident L0 L46.end
  constraint perpendicular L0 L46
  constraint coincident L0.end A2.end
  constraint perpendicular L48 L134
  constraint parallel L2 L49
  constraint parallel L2 L50
  constraint parallel L2 L51
  constraint parallel L51 L52
  constraint parallel L2 L53
  constraint parallel L2 L54
  constraint coincident L1.end L2.start
  constraint coincident L37 L56.end
  constraint perpendicular L37 L56
  constraint coincident L37 L57.end
  constraint perpendicular L37 L57
  constraint coincident L37 L120.end
  constraint perpendicular L37 L119
  constraint coincident L37 L122.end
  constraint perpendicular L37 L121
  constraint coincident L37 L113.end
  constraint perpendicular L37 L112
  constraint coincident L37 L116.end
  constraint perpendicular L37 L118
  constraint coincident L37 L129.end
  constraint perpendicular L37 L111
  constraint coincident L37 L127.end
  constraint perpendicular L37 L125
  constraint midpoint L58 L59.start
  constraint perpendicular L58 L59
  constraint symmetric L0.start L59 A19.end
  constraint symmetric L0.end L59 A21.start
  constraint symmetric A2.start L59 A21.end
  constraint symmetric A2 L59 A21
  constraint symmetric L1.end L59 L62.start
  constraint symmetric L6.end L59 L76.start
  constraint symmetric L7.end L59 L76.end
  constraint symmetric L8.end L59 A19.start
  constraint symmetric A4 L59 A19
  constraint symmetric A18 L59 A20
  constraint symmetric L34.end L59 L75.start
  constraint symmetric L35.end L59 L67.start
  constraint symmetric L39.end L59 L84.end
  constraint symmetric L36.end L59 L68.end
  constraint symmetric L37.end L59 L77.start
  constraint symmetric L38.end L59 L90.end
  constraint symmetric L39.start L59 L71.start
  constraint symmetric L41.end L59 L80.start
  constraint symmetric L42.end L59 L72.start
  constraint symmetric L43.start L59 L79.start
  constraint symmetric L43.end L59 L85.start
  constraint symmetric L44.end L59 L85.end
  constraint symmetric L124.end L59 L92.end
  constraint symmetric L123.end L59 L94.end
  constraint symmetric L115.end L59 L110.end
  constraint symmetric L114.end L59 L108.end
  constraint symmetric L46.end L59 L72.end
  constraint symmetric L48.end L59 L65.start
  constraint symmetric L49.end L59 L63.start
  constraint symmetric L50.end L59 L63.end
  constraint symmetric L51.end L59 L66.start
  constraint symmetric L52.end L59 L66.end
  constraint symmetric L53.end L59 L60.start
  constraint symmetric L54.end L59 L60.end
  constraint symmetric L56.end L59 L64.end
  constraint symmetric L57.end L59 L62.end
  constraint symmetric L120.end L59 L83.end
  constraint symmetric L122.end L59 L61.end
  constraint symmetric L113.end L59 L100.end
  constraint symmetric L116.end L59 L98.end
  constraint symmetric L129.end L59 L91.end
  constraint symmetric L127.end L59 L93.end
  constraint coincident L79 L91.start
  constraint collinear L91 L103
  constraint coincident L92.start L99
  constraint coincident L79 L93.start
  constraint collinear L93 L101
  constraint coincident L94.start L99
  constraint coincident A20 L102.end
  constraint coincident A20 L104.end
  constraint perpendicular L67 L95
  constraint coincident L72 L97.end
  constraint collinear L97 L98
  constraint coincident L72 L99.end
  constraint collinear L99 L100
  constraint coincident L72 L101.end
  constraint collinear L101 L102
  constraint coincident L72 L103.end
  constraint collinear L103 L104
  constraint perpendicular L84 L105
  constraint coincident A20 L109.start
  constraint coincident L100 L110.start
  constraint collinear L109 L110
  constraint coincident A20 L102.start
  constraint coincident L46 L111.end
  constraint collinear L111 L128
  constraint coincident L46 L112.end
  constraint collinear L112 L113
  constraint coincident L114.start L119
  constraint coincident L115.start L119
  constraint collinear L115 L117
  constraint collinear L116 L118
  constraint coincident L46 L118.end
  constraint coincident L46 L119.end
  constraint collinear L119 L120
  constraint coincident L46 L121.end
  constraint coincident L114 L122.start
  constraint collinear L121 L122
  constraint coincident L113 L124.start
  constraint coincident L46 L125.end
  constraint collinear L125 L126
  constraint coincident L45 L127.start
  constraint collinear L126 L127
  constraint coincident L45 L129.start
  constraint collinear L128 L129
  constraint coincident A18 L126.end
  constraint coincident A18 L128.end
  constraint coincident A18 L126.start
  constraint coincident A18 L117.start
  constraint coincident L130.end L132
  constraint perpendicular L130 L132
  constraint perpendicular L131 L132
  constraint collinear L132 L133
  constraint collinear L134 L135
  measures "d538" distance of L6.end L34.end
  measures "d539" distance of L34.end L35.end
  measures "d540" distance of L35.end L36.end
  measures "d541" distance of L36.end L38.end
  measures "d542" distance of L39.start L41.end
  measures "d543" distance of L41.end L42.end
  measures "d549" distance of L43.start L43.end
  measures "d550" angle of L44 L45
  measures "d551" distance of L39.start L48.end
  measures "d552" distance of L48.end L49.end
  measures "d553" distance of L49.end L50.end
  measures "d554" distance of L50.end L51.end
  measures "d555" distance of L51.end L52.end
  measures "d556" distance of L52.end L53.end
  measures "d557" distance of L53.end L54.end
extrude "Extrude69" add sketch "Sketch82" along normal blind 1 contours A0 | A1 | L0 L57 L123 L124 | L45 L56 L57 L124 | L56 L57 L123 L124 | L7 L8 L44 L45 L57 | L44 L45 L56 L57 | L0 L57 L114 L115 | L56 L57 L115 L123 | L56 L122 L123 L124 | L45 L56 L122 L124 | L44 L45 L56 L122 | L37 L44 L56 L57 | L0 L46 L57 L114 | L56 L57 L114 L115 | L56 L115 L122 L123 | L120 L122 L123 L124 | L45 L120 L122 L124 | L44 L45 L120 L122 | L37 L44 L56 L122 | L7 L35 L36 L37 L38 L40 L132 | L0 L46 L47 L57 | L46 L56 L57 L114 | L56 L114 L115 L122 | L115 L120 L122 L123 | L116 L120 L123 L124 | L45 L116 L120 L124 | L44 L45 L116 L120 | L37 L44 L120 L122 | L46 L47 L56 L57 | L2 L3 L4 L5 A3 L6 L7 L34 L35 L36 L45 L46 L56 L113 L114 L120 L123 L130 L131 L132 L133 | L114 L115 L120 L122 | L113 L116 L123 L124 | L45 L113 L116 L124 | L44 L45 L113 L116 | L1 L2 L47 L55 L56 L57 | L46 L47 L56 L121 | L44 L45 L113 L127 | L37 L44 L113 L116 | L2 L47 L54 L56 L121 | L46 L47 L119 L121 | L44 L45 L127 L129 | L37 L44 L113 L127 | L2 L47 L53 L119 L121 | L46 L47 L118 L119 | L43 L44 L45 L129 L134 | L37 L44 L127 L129 | L2 L47 L52 L118 L119 | L46 L47 L112 L118 | L2 L47 L51 L112 L118 | L46 L47 L112 L125 | L2 L47 L50 L112 L125 | L46 L47 L111 L125 | L2 L47 L49 L111 L125 | L42 L46 L47 L111 L135 | L2 L41 L47 L48 L111 L135 | L9 L10 L11 L12 | L13 L14 L15 A5 L16 A6 L17 A7 | L18 L19 L20 A8 L21 A9 L22 A10 | L23 L24 L25 A11 L27 A12 L28 A13 | L29 L30 L31 A14 L32 A15 L33 A16 | A17 | A18 L128 | A18 L126 L128 | A18 L117 L128 | A18 L126 | L61 L69 L80 L83 | L62 L64 L74 L80 L82 | L61 L72 L80 L83 | L61 L64 L72 L80 | L62 L64 L72 L80 | L61 L72 L83 L108 | L61 L64 L72 L108 | L72 L80 L83 L97 | L70 L80 L97 L99 | L62 L64 L72 L108 | L62 A21 L80 | L62 L72 L73 L80 | L61 L83 L108 L110 | L61 L64 L108 L110 | L72 L80 L97 L99 | L62 L64 L108 L110 | L62 L72 L73 L108 | L61 L83 L94 L110 | L83 L98 L108 L110 | L72 L80 L99 L101 | L65 L80 L101 L103 | L62 L64 L94 L110 | L62 L73 L108 L110 | L61 L83 L92 L94 | L61 L64 L92 L94 | L83 L94 L98 L110 | L98 L100 L108 L110 | L72 L80 L101 L103 | L71 L80 L81 L103 L107 | L62 L64 L92 L94 | L62 L73 L94 L110 | L61 L79 L83 L92 | L83 L92 L94 L98 | L94 L98 L100 L110 | L72 L80 L88 L103 L107 | L62 L64 L79 L92 | L62 L73 L92 L94 | L61 L79 L83 L85 | L61 L64 L79 L85 | L79 L83 L92 L98 | L92 L94 L98 L100 | L62 L64 L79 L85 | L62 A19 L73 L92 | L61 L83 L85 L89 | L79 L83 L85 L98 | L79 L92 L98 L100 | L62 L64 L85 L89 | L62 L76 L78 L79 L85 | L67 L68 L75 L76 L77 L89 L90 | L83 L85 L89 L98 | L79 L85 L98 L100 | L85 L89 L98 L100 | L79 L85 L93 L100 | L79 L85 L91 L93 | L85 L89 L91 L93 | L79 L85 L86 L91 L96 | L85 L89 L91 L96 | A20 L102 L104 | A20 L109 bodies 3